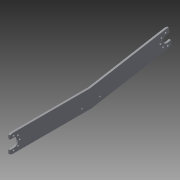
# Autodesk Inventor part: Arm_Link_1
Saved by Autodesk Inventor 2013 (Build 170138000, 138)
## iProperties
Created: 2014-05-15
Part Number: Arm_Link_1
Material: 一般
Document SubType Name: Modeling
Designer: andou
Density: 1 g/cm^3
Author: andou
Autodesk Inventor part; units mm, degrees
ref_plane "YZ Plane" through (0, 0, 0) normal (1, 0, 0) x (0, 1, 0)
ref_plane "XZ Plane" through (0, 0, 0) normal (0, 1, 0) x (-1, 0, 0)
ref_plane "XY Plane" through (0, 0, 0) normal (0, 0, 1) x (1, 0, 0)
sketch "スケッチ2" plane through (0, 0, 0) normal (1, 0, 0) x (0, 1, 0)
  line L0 (0, 0) -> (-84.4498, 0)
  line L1 (-84.4498, -20) -> (1.7498, -20)
  line L2 (0, 0) -> (83.1668, 14.6646)
  line L3 (86.6398, -5.0316) -> (1.7498, -20)
  arc A0 (87.251, 14.537) -> (83.1668, 14.6646) centre (84.9033, 4.8165) ccw
  arc A1 (86.6398, -5.0316) -> (90.434, -3.5148) centre (84.9033, 4.8165) ccw
  arc A2 (-88.4498, -19.1652) -> (-84.4498, -20) centre (-84.4498, -10) ccw
  arc A3 (-84.4498, 0) -> (-88.4498, -0.8348) centre (-84.4498, -10) ccw
  arc A4 (-84.4498, -15) -> (-84.4498, -5) centre (-84.4498, -10) ccw
  arc A5 (84.2087, 8.7557) -> (85.5979, 0.8772) centre (84.9033, 4.8165) ccw
  line L4 (84.2087, 8.7557) -> (88.1479, 9.4503)
  line L5 (85.5979, 0.8772) -> (89.5371, 1.5718)
  line L6 (-84.4498, -5) -> (-88.4498, -5)
  line L7 (-84.4498, -15) -> (-88.4498, -15)
  line L8 (-88.4498, -0.8348) -> (-88.4498, -5)
  line L9 (-88.4498, -15) -> (-88.4498, -19.1652)
  line L10 (87.251, 14.537) -> (88.1479, 9.4503)
  line L11 (89.5371, 1.5718) -> (90.434, -3.5148)
  line L12 (1.7498, -20) -> (0, 0)
  dimension "d21" = 20
  dimension "d22" = 10
  dimension "d23" = 170
  dimension "d25" = 10
  dimension "d27" = 10
  dimension "d31" = 10
  dimension "d32" = 8
  dimension "d33" = 4
  dimension "d35" = 4
  dimension "d36" = 170
  constraints: 26 end point, 12 perpendicular, 12 point on circle, 6 centre point, 4 equal length, 4 tangent, 3 equal radius, 2 coincident, 2 parallel, 1 horizontal
  measures "d21" distance between parallel lines of L0 L1
  measures "d22" distance from line of L0 A2.centre
  measures "d23" angle of L0 L2
  measures "d25" distance from line of L3 A0.centre
  measures "d27" radius of A3
  measures "d31" diameter of A4
  measures "d32" diameter of A5
  measures "d33" distance from line of L8 A2.centre
  measures "d35" distance from line of L10 L2.end
  measures "d36" distance of A2.centre A0.centre
extrude "押し出し1" add sketch "スケッチ2" along normal blind 2
sketch "スケッチ3" plane through (2, 0, 0) normal (1, 0, 0) x (0, 0, -1)
  arc A0 (0, -84.4498) -> (0.8348, -88.4498) centre (10, -84.4498) ccw projected
  line L0 (0.8348, -88.4498) -> (5, -88.4498) projected
  arc A1 (5.0316, 86.6398) -> (3.5148, 90.434) centre (-4.8165, 84.9033) ccw projected
  line L1 (3.5148, 90.434) -> (-1.5718, 89.5371) projected
  circle A2 centre (3, -84.4498) radius 1
  circle A3 centre (2.0772, 86.1188) radius 1
  dimension "d39" = 4
  dimension "d40" = 7
  dimension "d41" = 2
  dimension "d42" = 4
  dimension "d43" = 7
  constraints: 2 centre point, 1 equal radius
  measures "d39" distance from line of L0 A2.centre
  measures "d40" distance of A2.centre A0.centre
  measures "d41" diameter of A2
  measures "d42" distance from line of L1 A3.centre
  measures "d43" distance of A1.centre A3.centre
hole "穴1" at (2, 86.1188, -2.0772) at (2, -84.4498, -3) direction (-1, 0, 0) diameter 2 end through all
pattern_circular "円形状パターン1" count 5 over 180 about axis through (0, -84.4498, -10) along (-1, 0, 0) of "穴1"
pattern_circular "円形状パターン2" count 5 over 180 about axis through (0, 84.9033, 4.8165) along (-1, 0, 0) of "穴1"
sketch "スケッチ4" plane through (0, 0, 0) normal (-1, 0, 0) x (0, 0, 1)
  line L0 (-20, 1.7498) -> (-5.0316, 86.6398) projected
  line L1 (-20, -84.4498) -> (-20, 1.7498) projected
  circle A0 centre (-15, -8.7259) radius 1
  circle A1 centre (-13.2569, 11.198) radius 1
  line L2 (-15, -8.7259) -> (-13.2569, 11.198)
  dimension "d57" = 2
  dimension "d59" = 20
  dimension "d60" = 175
  dimension "d61" = 5
  dimension "d62" = 5
  constraints: 2 centre point, 2 end point, 1 equal radius
  measures "d57" diameter of A0
  measures "d59" distance of L2.start L2.end
  measures "d60" angle of L1 L2
  measures "d61" distance from line of L1 L2.start
  measures "d62" distance from line of L0 L2.end
hole "穴2" at (0, -8.7259, -15) at (0, 11.198, -13.2569) direction (1, 0, 0) diameter 1.6 end through all
